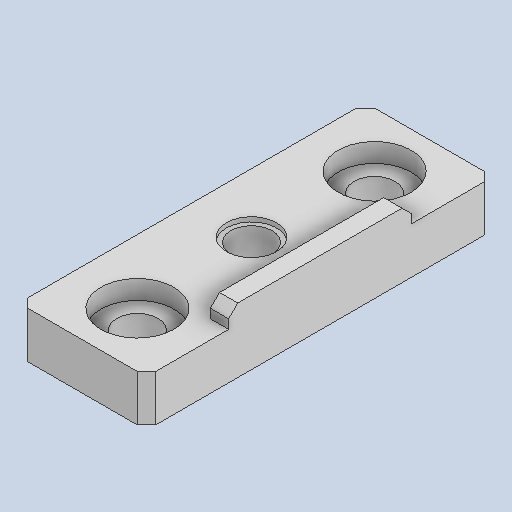
# Autodesk Inventor part: ADAPTER_RSP05-BH19.05
Saved by Autodesk Inventor 2024.2 (Build 282272000, 272)
## iProperties
ItemSpecifications: {"_id":"603fbadfb6e4f30009e2871c","finish":"543ef1f380da5b0c476373c1","finish_location":null,"material":"5515e170db035c20ce34af9a","process_initialism":null,"quotes":null,"current_quote":null,"quantity_ordered":1,"features":null,"hardware":null,"threading":null,"part_markings":[],"surface_roughness":null,"tolerance":null,"weld_quantity":null,"Notes":"","certifications":[],"part":null,"revision_num":0,"last_history":null,"inspection_requirement_details":{"inspection_requirement":"std","customer_data_sheet":null},"feedback":null}
Created: 2020-10-22
Part Number: ADAPTER_RSP05-BH19.05
Material: Generic
Document SubType Name: Modeling
Designer: qiti1
Density: 1 g/cm^3
Appearance: Default
Author: qiti1
Autodesk Inventor part; units mm, degrees
ref_plane "YZ Plane" through (0, 0, 0) normal (1, 0, 0) x (0, 1, 0)
ref_plane "XZ Plane" through (0, 0, 0) normal (0, 1, 0) x (-1, 0, 0)
ref_plane "XY Plane" through (0, 0, 0) normal (0, 0, 1) x (1, 0, 0)
sketch "Sketch1" plane through (0, 0, 0) normal (0, 1, 0) x (-1, 0, 0)
  line L0 (7, 10) -> (-7, 10)
  line L1 (-7, 10) -> (-7, -10)
  line L2 (-7, -10) -> (7, -10)
  line L3 (7, -10) -> (7, 10)
  line L4 (7, 10) -> (-7, -10) construction
  line L5 (-7, 10) -> (7, -10) construction
  point P0 (0, 0)
  dimension "POST_WIDTH" = 20
  dimension "POST_LENGTH" = 14
  constraints: 12 end point, 2 midpoint, 2 parallel, 1 horizontal, 1 perpendicular
  measures "POST_WIDTH" distance of L2.end L0.start
  measures "POST_LENGTH" distance of L1.end L2.end
extrude "Extrusion1" add sketch "Sketch1" along normal blind 5.075
sketch "Sketch2" plane through (0, 0, 0) normal (0, -1, 0) x (1, 0, 0)
  line L0 (-7, -19) -> (7, -19)
  line L1 (7, -19) -> (7, 19)
  line L2 (7, 19) -> (-7, 19)
  line L3 (-7, 19) -> (-7, -19)
  line L4 (-7, -19) -> (7, 19) construction
  line L5 (7, -19) -> (-7, 19) construction
  line L6 (-7, -10) -> (-7, 10) projected
  line L7 (-7, 10) -> (7, 10) projected
  point P0 (0, 0)
  dimension "d4" = 0
  dimension "WING_LENGTH" = 9
  constraints: 12 end point, 2 midpoint, 2 parallel, 1 horizontal, 1 perpendicular
  measures "d4" distance between parallel lines of L6 L3
  measures "WING_LENGTH" distance between parallel lines of L2 L7
extrude "Extrusion2" add sketch "Sketch2" against normal blind 5.075
sketch "Sketch3" plane through (0, 5.075, 0) normal (0, 1, 0) x (1, 0, 0)
  line L0 (-7, 19) -> (7, 19) projected
  line L1 (0, 19) -> (0, -19)
  line L2 (7, -19) -> (-7, -19) projected
  line L3 (7, 0) -> (-7, 0)
  line L4 (-7, -19) -> (-7, 19) projected
  point P0 (0, 0)
  point P1 (0, -13)
  point P2 (0, 13)
  dimension "d15" = 0
  dimension "d16" = 6
  constraints: 4 end point, 3 midpoint, 1 symmetric about line
  measures "d15" distance from line of L1 point (0, -13)
  measures "d16" distance from line of L2 point (0, -13)
hole "Hole1" at (0, 5.075, 13) at (0, 5.075, -13) direction (0, -1, 0) diameter 4.5 end through all counterbore diameter 8 counterbore depth 2.075 clearance for "Socket Head Cap Screw" size "#8" standard "Ansi Unified Screw Threads"
chamfer "Chamfer4" distance 1 angle 45 4 edges at (-7, 2.5375, 19) (7, 2.5375, 19) (-7, 2.5375, -19) (7, 2.5375, -19)
sketch "Sketch4" plane through (0, 5.075, 0) normal (0, 1, 0) x (1, 0, 0)
  line L0 (7, 10) -> (5, 10)
  line L1 (5, 10) -> (5, -10)
  line L2 (5, -10) -> (7, -10)
  line L3 (7, -10) -> (7, 10)
  line L4 (7, -18) -> (7, 18) projected
  point P0 (0, 0)
  dimension "d56" = 20
  dimension "d57" = 2
  dimension "d58" = 0
  dimension "d59" = 10
  constraints: 8 end point, 2 parallel, 1 horizontal, 1 perpendicular
  measures "d56" distance of L2.end L0.start
  measures "d57" distance of L1.end L2.end
  measures "d58" distance between parallel lines of L4 L3
  measures "d59" distance from line of point (0, 0) L2
extrude "Extrusion3" add sketch "Sketch4" along normal blind 2
sketch "Sketch5" plane through (0, 0, 0) normal (0, -1, 0) x (1, 0, 0)
  line L0 (-9.8, 0) -> (9.8, 0) projected
  line L1 (0, 26.6) -> (0, -26.6) projected
  line L2 (-7, 19) -> (-7, -19) projected
  line L3 (7, -10) -> (7, -18) projected
  line L4 (6, -19) -> (7, -18) projected
  line L5 (6, -19) -> (-6, -19) projected
  line L6 (-7, -18) -> (-6, -19) projected
  line L7 (-7, -18) -> (-7, 18) projected
  line L8 (-6, 19) -> (-7, 18) projected
  line L9 (-6, 19) -> (6, 19) projected
  line L10 (7, 18) -> (6, 19) projected
  line L11 (5, -10) -> (7, -10) projected
  line L12 (7, 18) -> (7, 10) projected
  line L13 (7, 10) -> (5, 10) projected
  line L14 (5, 10) -> (5, -10) projected
  point P0 (-0.5, 0)
hole "Hole2" at (-0.5, 0, 0) direction (0, 1, 0) diameter 4.5 end through all clearance for "Socket Head Cap Screw" size "#8" standard "Ansi Unified Screw Threads"
chamfer "Chamfer1" distance 1 angle 45 2 edges at (6, 7.075, -10) (6, 7.075, 10)
chamfer "Chamfer2" [suppressed]
sketch "Sketch7" plane through (0, 5.075, 0) normal (0, 1, 0) x (1, 0, 0)
  circle A0 centre (-0.5, 0) radius 2.75
  circle A1 centre (-0.5, 0) radius 2.25 projected
  point P0 (0, 0)
  dimension "d46" = 5.5
  constraints: 1 centre point, 1 concentric
  measures "d46" diameter of A0
extrude "Extrusion5" cut sketch "Sketch7" against normal blind 0.5 contours A0 | A1
equation "\"POST_LENGTH\" = 2 * LIP_THICKNESS + BASE_THICKNESS"
equation "\"POST_HEIGHT\" = BEAM_HEIGHT - BASE2APERTURE_CENTER"
equation "\"BASE2APERTURE_CENTER\" = 13.975"
equation "\"BEAM_HEIGHT\" = 19.05"
equation "\"WALL_GAP\" = 0.5"
equation "\"LIP_THICKNESS\" = 2"
equation "\"BASE_THICKNESS\" = 10"
body "Solid1"
